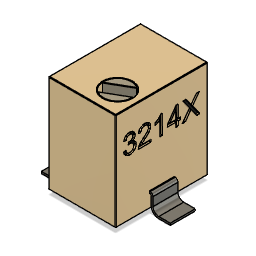
Bourns 3214X v3 (Autodesk Fusion 360 design; units mm, degrees)
Autodesk Fusion 360 part; units mm, degrees
sketch "Sketch1" plane through (0, 0, 0) normal (0, 1, 0) x (1, 0, 0) in component "Resistor Body"
  line L0 (-1.75, -2.4) -> (1.75, -2.4)
  line L1 (1.75, -2.4) -> (1.75, 2.4)
  line L2 (1.75, 2.4) -> (-1.75, 2.4)
  line L3 (-1.75, 2.4) -> (-1.75, -2.4)
  line L4 (0, 2.4) -> (0, -2.4) construction
  dimension "d1" = 3.5
  dimension "d2" = 4.8
  constraint horizontal L0
  constraint vertical L1
  constraint horizontal L2
  constraint vertical L3
  constraint midpoint L2 L4.start
  constraint midpoint L0 L4.end
  constraint midpoint origin L4
  measures "d1" distance of L1.end L2.end
  measures "d2" distance of L0.end L1.end
extrude "Extrude1" add sketch "Sketch1" along normal blind 5.1 makes body 1 in component "Resistor Body"
sketch "Sketch1 (1)" plane through (0, 5.1, 0) normal (0, 1, 0) x (-1, 0, 0) in component "Resistor Body"
  line L0 (1.75, -2.4) -> (1.75, 2.4)
  line L1 (1.75, 2.4) -> (-1.75, 2.4)
  line L2 (-1.75, 2.4) -> (-1.75, -2.4)
  line L3 (-1.75, -2.4) -> (1.75, -2.4)
  circle A0 centre (-0.65, 1.2) radius 0.75
  dimension "d5" = 1.5
  dimension "d6" = 2.4
  dimension "d8" = 1.2
  measures "d5" diameter of A0
  measures "d6" distance of L0 A0.centre
  measures "d8" vertical distance of origin A0.centre
extrude "Extrude1'" cut sketch "Sketch1 (1)" against normal blind 1 contours A0 bodies 1 in component "Resistor Body"
sketch "Sketch2" plane through (1.75, 0, 0) normal (1, 0, 0) x (0, 0, -1) in component "Resistor Body"
  line L0 (-2.4, 0) -> (2.4, 0)
  line L1 (2.4, 0) -> (2.4, 5.1)
  line L2 (2.4, 5.1) -> (-2.4, 5.1)
  line L3 (-2.4, 5.1) -> (-2.4, 0)
  line L4 (-1.8074, 2.9881) -> (1.8143, 3.0119) construction
  line L5 (1.8143, 3.0119) -> (1.8081, 3.9547) construction
  line L6 (1.8081, 3.9547) -> (-1.8136, 3.931) construction
  line L7 (-1.8136, 3.931) -> (-1.8074, 2.9881) construction
  dimension "d11" = 3
  text T0 "3214X" font "Arial" height 1 align centre middle in box 3.6218 x 0.9429 at (-1.8074, 2.9881) x (0.999979, 0.006545) y (-0.006545, 0.999979) spacing 1
  measures "d11" distance of origin
extrude "Extrude2" cut sketch "Sketch2" against normal blind 0.1 text T0 bodies 1 in component "Resistor Body"
sketch "Sketch1 (2)" plane through (0, 4.1, 0) normal (0, 1, 0) x (-1, 0, 0) in component "Adjustment"
  circle A0 centre (-0.65, 1.2) radius 0.75
  circle A1 centre (-0.65, 1.2) radius 0.745
  dimension "d14" = 1.49
  constraint concentric A0 A1
  measures "d14" diameter of A1
extrude "Extrude1''" add sketch "Sketch1 (2)" along normal up to surface (1 mm away) separate body contours A1 makes body 2 in component "Adjustment"
sketch "Sketch2 (2)" plane through (0, 5.1, 0) normal (0, 1, 0) x (-1, 0, 0) in component "Adjustment"
  circle A0 centre (-0.65, 1.2) radius 0.745
  line L0 (0.1495, 1.3152) -> (-1.1495, 0.5652)
  line L1 (-1.1495, 0.5652) -> (-1.4495, 1.0848)
  line L2 (-1.4495, 1.0848) -> (-0.1505, 1.8348)
  line L3 (-0.1505, 1.8348) -> (0.1495, 1.3152)
  line L4 (-0.0005, 1.575) -> (-1.2995, 0.825) construction
  line L5 (-0.65, 1.2) -> (-0.65, 0.455) construction
  dimension "d17" = 0.6
  dimension "d18" = 120
  dimension "d19" = 1.5
  constraint midpoint L3 L4.start
  constraint midpoint L1 L4.end
  constraint midpoint A0.centre L4
  constraint coincident A0.centre L5.start
  constraint coincident A0 L5.end
  constraint perpendicular L0 L3
  constraint perpendicular L2 L3
  constraint perpendicular L1 L2
  constraint vertical L5
  measures "d17" distance of L0.start L2.end
  measures "d18" angle of L4 L5
  measures "d19" distance of L1.end L2.end
extrude "Extrude2'" cut sketch "Sketch2 (2)" against normal blind 0.5 contours A0 L0 L2 bodies 2 in component "Adjustment"
sketch "Sketch3" plane through (0, 0, 2.4) normal (0, 0, 1) x (1, 0, 0) in component "Leads"
  line L0 (-1.75, 0) -> (1.75, 0)
  line L1 (1.75, 0) -> (1.75, 5.1)
  line L2 (1.75, 5.1) -> (-1.75, 5.1)
  line L3 (-1.75, 5.1) -> (-1.75, 0)
  line L4 (1.75, 0) -> (1.75, 0.8) construction
  line L5 (1.75, 0.7) -> (1.8, 0.7)
  line L6 (1.85, 0.65) -> (1.85, 0.2)
  line L7 (2.25, -0.2) -> (2.85, -0.2)
  line L8 (2.85, -0.2) -> (2.85, -0.1)
  line L9 (2.85, -0.1) -> (2.25, -0.1)
  line L10 (1.95, 0.2) -> (1.95, 0.65)
  line L11 (1.8, 0.8) -> (1.75, 0.8)
  line L12 (1.75, 0.7) -> (1.75, 0.8) construction
  arc A0 (1.85, 0.65) -> (1.8, 0.7) centre (1.8, 0.65) ccw
  arc A1 (1.95, 0.65) -> (1.8, 0.8) centre (1.8, 0.65) ccw
  arc A2 (1.85, 0.2) -> (2.25, -0.2) centre (2.25, 0.2) ccw
  arc A3 (1.95, 0.2) -> (2.25, -0.1) centre (2.25, 0.2) ccw
  point P0 (1.95, 0.8)
  dimension "d22" = 0.8
  dimension "d23" = 0.1
  dimension "d24" = 0.1
  dimension "d25" = 0.1
  dimension "d26" = 5.3
  dimension "d27" = 0.2
  dimension "d28" = 0.05
  dimension "d31" = 0.3
  dimension "d32" = 1
  constraint coincident L0.end L1.start
  constraint coincident L1 L4.end
  constraint coincident L4 L5.start
  constraint perpendicular L1 L5
  constraint perpendicular L5 L6
  constraint perpendicular L1 L7
  constraint perpendicular L5 L8
  constraint perpendicular L1 L9
  constraint perpendicular L9 L10
  constraint tangent L5 A0
  constraint tangent L6 A0
  constraint coincident P0 L11
  constraint coincident P0 L10
  constraint tangent L11 A1
  constraint tangent L10 A1
  constraint coincident A0.centre A1.centre
  constraint tangent L6 A2
  constraint tangent L7 A2
  constraint tangent L10 A3
  constraint tangent L9 A3
  constraint coincident A2.centre A3.centre
  measures "d22" distance of L0.end L4.end
  measures "d23" distance of L6 L10
  measures "d24" distance of L5 L11
  measures "d25" distance of L7 L9
  measures "d26" vertical distance of L1.end L7.end
  measures "d27" distance of L1 P0
  measures "d28" radius of A0
  measures "d31" radius of A3
  measures "d32" distance of L6 L7.end
extrude "Extrude1'''" add sketch "Sketch3" along normal blind 1.3 separate body contours L1 L5 L6 L7 L8 L9 L10 L11 A0 A1 A2 A3 makes body 3 in component "Leads"
move_body "Move1" bodies 3 to x (1, 0, 0) y (0, 1, 0) z (0, 0, 1) at (0, 0, -3.1) in component "Leads"
move_body "Move2" bodies 3 to x (1, 0, 0) y (0, 1, 0) z (0, 0, 1) at (0, 0, 0.05) in component "Leads"
copy_body "CopyPasteBodies1" bodies 3 makes body 4 in component "Leads"
move_body "Move3" bodies 4 to x (-1, 0, 0) y (0, 1, 0) z (0, 0, -1) at (-0.1, 0, 2.1) in component "Leads"
extrude "Extrude2''" cut 1 faces at (-2.55, -0.1333, 2.75) along direction (0, 0, -1) blind 0.5 on bodies 4 bodies 4 in component "Leads"
move_body "Move4" bodies 4 to x (1, 0, 0) y (0, 1, 0) z (0, 0, 1) at (0, 0, -0.8) in component "Leads"
copy_body "CopyPasteBodies2" bodies 4 makes body 5 in component "Leads"
move_body "Move5" bodies 5 to x (1, 0, 0) y (0, 1, 0) z (0, 0, 1) at (0, 0, -2.54) in component "Leads"
move_body "Move6" bodies 4 5 to x (1, 0, 0) y (0, 1, 0) z (0, 0, 1) at (0, 0, 0.205) in component "Leads"
move_body "Move7" bodies 4 5 to x (1, 0, 0) y (0, 1, 0) z (0, 0, 1) at (0, 0, 0.015) in component "Leads"
sketch "Sketch1 (3)" plane through (0, 0, 0) normal (0, 0, 1) x (1, 0, 0) in component "Leads"
fillet "Fillet1" radius 0.02 4 edges at (0.5, 5.1, 0.9402) (0.5, 4.6, 0.9402) (0.8, 5.1, 1.4598) (0.8, 4.6, 1.4598) on bodies 2 in component "Adjustment"
fillet "Fillet1'" radius 0.03 13 edges at (1.3492, 5.1, 1.4712) (1.75, 5.1, 0) (0, 5.1, 2.4) (1.75, 2.55, 2.4) (-1.75, 2.55, 2.4) (1.75, 2.55, -2.4) (0, 5.1, -2.4) (-1.75, 2.55, -2.4) (0, 0, -2.4) (-1.75, 0, 0) (0, 0, 2.4) (1.75, 0, 0) (-1.75, 5.1, 0) on bodies 1 in component "Resistor Body"
fillet "Fillet2" radius 0.02 16 edges at (1.0851, 5.0945, 0.5953) (1.0906, 4.85, 0.5992) (1.0959, 4.6056, 0.6032) (1.2952, 4.6, 0.8275) (1.3898, 4.6056, 1.1122) (1.3906, 4.85, 1.1188) (1.3913, 5.0945, 1.1256) (1.0225, 5.1, 1.8452) (0.2149, 5.0945, 1.8047) (0.2094, 4.85, 1.8008) (0.2041, 4.6056, 1.7968) (0.0048, 4.6, 1.5725) (-0.0898, 4.6056, 1.2878) (-0.0906, 4.85, 1.2812) (-0.0913, 5.0945, 1.2744) (0.2775, 5.1, 0.5548) on bodies 2 in component "Adjustment"
move_body "Move8" bodies 5 4 to x (1, 0, 0) y (0, 1, 0) z (0, 0, 1) at (0.1, 0, 0) in component "Leads"
extrude "Extrude3" [suppressed] in component "Leads"
component "Resistor Body" placed x (1, 0, 0) y (0, 1, 0) z (0, 0, 1) at (0, 0, 0)
component "Leads" placed x (1, 0, 0) y (0, 1, 0) z (0, 0, 1) at (0, 0, 0)
component "Adjustment" placed x (1, 0, 0) y (0, 1, 0) z (0, 0, 1) at (0, 0, 0) in component "Resistor Body"
equation "d24 = d23"
equation "d25 = d23"
named bodies: "Lead 2", "Lead 3", "Lead 1"
